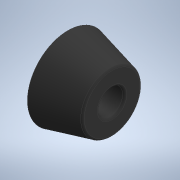
# Autodesk Inventor part: Rubberfoot
Saved by Autodesk Inventor 2020.2 (Build 242310000, 310)
## iProperties
Created: 2020-08-24
Part Number: Rubberfoot
Material: Generic
Document SubType Name: Modeling
Designer: JK
Density: 1 g/cm^3
Appearance: Rubber - Black
Author: JK
Autodesk Inventor part; units mm, degrees
ref_plane "YZ Plane" through (0, 0, 0) normal (1, 0, 0) x (0, 1, 0)
ref_plane "XZ Plane" through (0, 0, 0) normal (0, 1, 0) x (-1, 0, 0)
ref_plane "XY Plane" through (0, 0, 0) normal (0, 0, 1) x (1, 0, 0)
sketch "Sketch2" plane through (0, 0, 0) normal (0, 1, 0) x (-1, 0, 0)
  line L0 (0, 0) -> (0, -14)
  line L1 (0, -14) -> (21, -19.25)
  line L2 (21, -19.25) -> (21, 0)
  line L3 (21, 0) -> (0, 0)
  dimension "d1" = 14
  dimension "d2" = 21
  dimension "d3" = 19.25
  constraints: 8 end point, 2 vertical, 1 perpendicular
  measures "d1" distance of L0.start L0.end
  measures "d2" distance between parallel lines of L2 L0
  measures "d3" distance of L1.end L2.end
revolve "Revolution1" add sketch "Sketch2" angle 360 about axis through (-21, 0, 0) along (1, 0, 0)
sketch "Sketch3" plane through (-21, 0, 0) normal (-1, 0, 0) x (0, 0, 1)
  circle A0 centre (0, 0) radius 3
  dimension "d5" = 6
  constraints: 1 centre point, 1 coincident
  measures "d5" diameter of A0
extrude "Extrusion1" cut sketch "Sketch3" against normal through all
sketch "Sketch4" plane through (0, 0, 0) normal (1, 0, 0) x (0, 0, -1)
  circle A0 centre (0, 0) radius 6
  dimension "d8" = 12
  constraints: 1 centre point, 1 coincident
  measures "d8" diameter of A0
extrude "Extrusion2" cut sketch "Sketch4" against normal blind 10.5
fillet "Fillet1" radius 1 2 edges at (0, 0, 14) (0, 0, 6)
body "Solid1"
